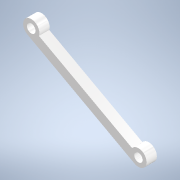
# Autodesk Inventor part: palanca base_proxima
Saved by Autodesk Inventor 2020.4 (Build 244396010, 396A)
## iProperties
Created: 2021-08-20
Part Number: palanca base_proxima
Material: PPS Plastic
Document SubType Name: Modeling
Designer: chalo
Density: 1.637 g/cm^3
Appearance: Smooth - White
Author: chalo
Autodesk Inventor part; units mm, degrees
ref_plane "YZ Plane" through (0, 0, 0) normal (1, 0, 0) x (0, 1, 0)
ref_plane "XZ Plane" through (0, 0, 0) normal (0, 1, 0) x (-1, 0, 0)
ref_plane "XY Plane" through (0, 0, 0) normal (0, 0, 1) x (1, 0, 0)
sketch "Sketch1" plane through (0, 0, 0) normal (0, 0, 1) x (1, 0, 0)
  circle A0 centre (-25.35, -26.8891) radius 1.55 projected
  circle A1 centre (-25.35, -26.8891) radius 3
  circle A2 centre (-64.85, -5.4402) radius 1.6 projected
  circle A3 centre (-64.85, -5.4402) radius 3
  line L0 (-26.7816, -29.5255) -> (-66.2816, -8.0766) construction
  line L1 (-23.9184, -24.2527) -> (-63.4184, -2.8038) construction
  line L2 (-26.7816, -29.5255) -> (-45.35, -19.4427)
  line L3 (-62.0119, -6.4124) -> (-62.0119, -6.4124)
  line L4 (-32.35, -16.7754) -> (-65.35, -16.7754)
  line L5 (-32.35, -5.7754) -> (-57.816, -5.7754)
  line L6 (-32.35, -5.7754) -> (-32.35, -16.7754) construction
  line L7 (-32.35, -11.2754) -> (-52.35, -11.2754) construction
  line L8 (-63.35, -12.7754) -> (-63.35, -16.4711) construction
  line L9 (-45.35, -19.4427) -> (-66.2816, -8.0766)
  line L10 (-62.0119, -6.4124) -> (-27.7109, -25.0381)
  point P0 (0, 0)
  point P1 (-47.8172, -11.2754)
  dimension "d0" = 6
  dimension "d1" = 6
  dimension "d10" = 20
  dimension "d11" = 20
  dimension "d19" = 3.5
  constraints: 20 end point, 7 point on circle, 5 tangent, 3 horizontal, 3 point on line, 2 centre point, 2 coincident, 1 midpoint, 1 vertical, 4 other
  measures "d0" diameter of A1
  measures "d1" diameter of A3
  measures "d10" horizontal distance of A0.centre L2.end
  measures "d11" distance of L7.start L7.end
  measures "d19" distance between parallel lines of L10 L0
extrude "Extrusion1" add sketch "Sketch1" along normal mid plane 3.8
body "Solid1"
